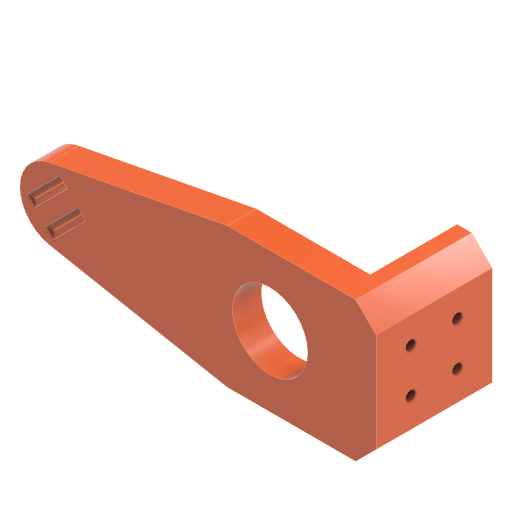
# Autodesk Inventor part: Corner Z Axis Carriage
Saved by Autodesk Inventor 2023.2 (Build 272271000, 271)
## iProperties
Created: 2023-02-17
Part Number: Corner Z Axis Carriage
Material: ABS Plastic
Document SubType Name: Modeling
Designer: remop
Density: 1.06 g/cm^3
Appearance: Smooth - Light Orange
Author: remop
Autodesk Inventor part; units mm, degrees
ref_plane "YZ Plane" through (0, 0, 0) normal (1, 0, 0) x (0, 1, 0)
ref_plane "XZ Plane" through (0, 0, 0) normal (0, 1, 0) x (-1, 0, 0)
ref_plane "XY Plane" through (0, 0, 0) normal (0, 0, 1) x (1, 0, 0)
sketch "Sketch1" plane through (0, 0, 0) normal (0, 0, 1) x (1, 0, 0)
  arc A0 (18.184259, -16.532371) -> (18.761762, -13.100955) centre (16.062938, -14.41105) ccw
  arc A1 (18.761762, 13.100955) -> (18.761762, -13.100955) centre (45.75, 0) ccw
  arc A2 (18.761762, 13.100955) -> (18.184259, 16.532371) centre (16.062938, 14.41105) ccw
  line L0 (11.532371, 23.184259) -> (18.184259, 16.532371)
  arc A3 (11.532371, 23.184259) -> (8.100955, 23.761762) centre (9.41105, 21.062938) ccw
  arc A4 (-18.100955, 23.761762) -> (8.100955, 23.761762) centre (-5, 50.75) ccw
  arc A5 (-18.100955, 23.761762) -> (-21.532371, 23.184259) centre (-19.41105, 21.062938) ccw
  line L1 (-28.184259, 16.532371) -> (-21.532371, 23.184259)
  arc A6 (-28.184259, 16.532371) -> (-28.761762, 13.100955) centre (-26.062938, 14.41105) ccw
  arc A7 (-28.761762, -13.100955) -> (-28.761762, 13.100955) centre (-55.75, 0) ccw
  arc A8 (-28.761762, -13.100955) -> (-28.184259, -16.532371) centre (-26.062938, -14.41105) ccw
  line L2 (-21.532371, -23.184259) -> (-28.184259, -16.532371)
  arc A9 (-21.532371, -23.184259) -> (-18.100955, -23.761762) centre (-19.41105, -21.062938) ccw
  arc A10 (8.100955, -23.761762) -> (-18.100955, -23.761762) centre (-5, -50.75) ccw
  arc A11 (8.100955, -23.761762) -> (11.532371, -23.184259) centre (9.41105, -21.062938) ccw
  line L3 (18.184259, -16.532371) -> (11.532371, -23.184259)
  circle A12 centre (10, -15) radius 4
  circle A13 centre (-20, -15) radius 4
  circle A14 centre (-20, 15) radius 4
  circle A15 centre (10, 15) radius 4
  circle A16 centre (-5, 0) radius 13
  line L4 (39.464466, -4.5) -> (34.964466, -4.5)
  line L5 (34.964466, -4.5) -> (34.964466, 4.5)
  line L6 (34.964466, 4.5) -> (39.464466, 4.5)
  line L7 (39.464466, 4.5) -> (39.464466, 10)
  line L8 (39.464466, 10) -> (31.464466, 10)
  line L9 (31.464466, 10) -> (31.464466, -10)
  line L10 (31.464466, -10) -> (39.464466, -10)
  line L11 (39.464466, -10) -> (39.464466, -4.5)
  line L12 (31.464466, -10) -> (31.464466, -17.071068)
  line L13 (31.464466, -17.071068) -> (24.472595, -24.062938)
  line L14 (31.464466, 10) -> (31.464466, 17.071068)
  line L15 (-19.41105, -24.062938) -> (24.472595, -24.062938)
  line L16 (-19.41105, 24.062938) -> (24.472595, 24.062938)
  line L17 (31.464466, 17.071068) -> (24.472595, 24.062938)
  circle A17 centre (-78.5, 0) radius 12.5
  line L18 (-19.978787, -24.008728) -> (-80.865571, -12.274122)
  line L19 (-80.865571, 12.274122) -> (-19.978787, 24.008728)
  point P0 (0, 0)
  dimension "d0" = 45
  dimension "d1" = 5
  dimension "d4" = 78.5
  dimension "d5" = 25
  constraints: 16 end point, 8 tangent, 6 point on circle, 3 equal length, 2 vertical, 1 centre point, 1 horizontal alignment, 1 point on line
  measures "d0" angle of L12 L13
  measures "d1" distance from line of L9.end L13
  measures "d4" distance of A17.centre point (0, 0)
  measures "d5" diameter of A17
extrude "Extrusion1" add sketch "Sketch1" along normal blind 10 contours L3 A11 A10 A9 L2 A8 A7 A6 L1 A5 A4 A3 L0 A2 A1 A0 | A0 A1 A2 L0 A3 L16 L17 L14 L9 L12 L13 L15 A11 L3 | L15 A9 A10 A11 | L18 A17 L19 A5 L1 A6 A7 A8 L2 A9 | A3 A4 A5 L16 | A17 | A12 | A14
sketch "Sketch2" plane through (0, 0, 0) normal (0, 0, -1) x (-1, 0, 0)
  line L0 (-24.472595, -24.062938) -> (-31.464466, -17.071068)
  line L1 (19.41105, -24.062938) -> (-24.472595, -24.062938)
  arc A0 (19.41105, -24.062938) -> (19.978787, -24.008728) centre (19.41105, -21.062938) ccw
  line L2 (80.865571, -12.274122) -> (19.978787, -24.008728)
  arc A1 (80.865571, -12.274122) -> (80.865571, 12.274122) centre (78.5, 0) ccw
  line L3 (19.978787, 24.008728) -> (80.865571, 12.274122)
  arc A2 (19.978787, 24.008728) -> (19.41105, 24.062938) centre (19.41105, 21.062938) ccw
  line L4 (-24.472595, 24.062938) -> (19.41105, 24.062938)
  line L5 (-31.464466, 17.071068) -> (-24.472595, 24.062938)
  line L6 (-31.464466, -17.071068) -> (-31.464466, 17.071068)
  circle A3 centre (20, -15) radius 4
  circle A4 centre (-10, 15) radius 4
  circle A5 centre (5, 0) radius 13
  line L7 (-31.464466, 17.071068) -> (-23.464466, 17.071068)
  line L8 (-23.464466, 17.071068) -> (-23.464466, -17.071068)
  line L9 (-24.472595, -24.062938) -> (-31.464466, -17.071068)
  line L10 (-23.464466, -17.071068) -> (-31.464466, -17.071068)
  line L11 (-23.464466, 17.071068) -> (-19.472595, 21.062938)
  line L12 (-19.472595, 21.062938) -> (-19.472595, 24.062938)
  line L13 (-23.464466, -17.071068) -> (-19.472595, -21.062938)
  line L14 (-19.472595, -21.062938) -> (-19.472595, -24.062938)
  line L15 (19.41105, -24.062938) -> (-24.472595, -24.062938)
  point P0 (0, 0)
  dimension "d6" = 8
  dimension "d9" = 3
  constraints: 14 end point, 3 perpendicular, 3 point on line, 2 horizontal, 1 parallel, 1 vertical
  measures "d6" distance of L5.start L7.end
  measures "d9" distance of L11.end L12.end
extrude "Extrusion2" add sketch "Sketch2" along normal blind 29.9 contours L0 L10 L13 L14 L1 | L6 L7 L8 L10 | L5 L4 L12 L11 L7
sketch "Sketch3" plane through (23.464466, -17.071068, 0) normal (-1, 0, 0) x (0, 0, 1)
  line L0 (0, 34.142136) -> (0, 0)
  line L1 (0, 34.142136) -> (-29.9, 34.142136)
  line L2 (-29.9, 0) -> (-29.9, 34.142136)
  line L3 (0, 0) -> (-29.9, 0)
  point P0 (0, 17.071068)
  point P1 (-1.95, 25.015758)
  point P2 (-17.95, 25.015758)
  point P3 (-17.95, 10.015758)
  point P4 (-1.95, 10.015758)
  dimension "d10" = 15
  dimension "d11" = 16
  dimension "d12" = 11.95
  constraints: 2 horizontal alignment, 2 vertical alignment
  measures "d10" distance of point (-1.95, 10.016) point (-1.95, 25.016)
  measures "d11" distance of point (-17.95, 25.016) point (-1.95, 25.016)
  measures "d12" distance from line of L2 point (-17.95, 25.016)
hole "Hole1" at (23.464466, 7.94469, -1.95) at (23.464466, 7.94469, -17.95) at (23.464466, -7.05531, -17.95) at (23.464466, -7.05531, -1.95) direction (1, 0, 0) diameter 3.6 end through all counterbore diameter 6.5 counterbore depth 3.4 clearance for "Socket Head Cap Screw DIN EN ISO 4762" size "M3" standard "DIN"
sketch "Sketch4" plane through (0, 0, 0) normal (0, 0, -1) x (-1, 0, 0)
  circle A0 centre (5, 0) radius 13
  circle A1 centre (-10, 15) radius 4
  circle A2 centre (20, -15) radius 4
  line L0 (-19.472595, 24.062938) -> (-19.472595, 21.062938)
  line L1 (-19.472595, 21.062938) -> (-23.464466, 17.071068)
  line L2 (-23.464466, 17.071068) -> (-23.464466, 10.54469)
  line L3 (-23.464466, 10.54469) -> (-23.464466, 5.34469)
  line L4 (-23.464466, 5.34469) -> (-23.464466, -4.45531)
  line L5 (-23.464466, -4.45531) -> (-23.464466, -9.65531)
  line L6 (-23.464466, -9.65531) -> (-23.464466, -17.071068)
  line L7 (-23.464466, -17.071068) -> (-19.472595, -21.062938)
  line L8 (-19.472595, -21.062938) -> (-19.472595, -24.062938)
  line L9 (19.41105, -24.062938) -> (-19.472595, -24.062938)
  arc A3 (19.41105, -24.062938) -> (19.978787, -24.008728) centre (19.41105, -21.062938) ccw
  line L10 (80.865571, -12.274122) -> (19.978787, -24.008728)
  arc A4 (80.865571, -12.274122) -> (80.865571, 12.274122) centre (78.5, 0) ccw
  line L11 (19.978787, 24.008728) -> (80.865571, 12.274122)
  arc A5 (19.978787, 24.008728) -> (19.41105, 24.062938) centre (19.41105, 21.062938) ccw
  line L12 (-19.472595, 24.062938) -> (19.41105, 24.062938)
  line L13 (-19.472595, 21.062938) -> (-15.480725, 17.071068)
  line L14 (-15.480725, 17.071068) -> (-15.480725, -17.071068)
  line L15 (-15.480725, -17.071068) -> (-19.472595, -21.062938)
  line L16 (-23.464466, 17.071068) -> (-19.472595, 21.062938)
  point P0 (0, 0)
  constraints: 6 end point, 3 perpendicular, 1 vertical
extrude "Extrusion3" cut sketch "Sketch4" against normal blind 2 contours L13 L14 L15 L7 L6 L5 L4 L3 L2 L1
sketch "Sketch5" plane through (0, 0, 10) normal (0, 0, 1) x (1, 0, 0)
  line L0 (24.472595, -24.062938) -> (31.464466, -17.071068)
  line L1 (31.464466, -17.071068) -> (31.464466, 17.071068)
  line L2 (31.464466, 17.071068) -> (24.472595, 24.062938)
  line L3 (24.472595, 24.062938) -> (-19.41105, 24.062938)
  arc A0 (-19.41105, 24.062938) -> (-19.978787, 24.008728) centre (-19.41105, 21.062938) ccw
  line L4 (-19.978787, 24.008728) -> (-80.865571, 12.274122)
  arc A1 (-80.865571, 12.274122) -> (-80.865571, -12.274122) centre (-78.5, 0) ccw
  line L5 (-80.865571, -12.274122) -> (-19.978787, -24.008728)
  arc A2 (-19.978787, -24.008728) -> (-19.41105, -24.062938) centre (-19.41105, -21.062938) ccw
  line L6 (-19.41105, -24.062938) -> (24.472595, -24.062938)
  circle A3 centre (-20, -15) radius 4
  circle A4 centre (10, 15) radius 4
  circle A5 centre (-5, 0) radius 13
  line L7 (-88.753048, -1.06066) -> (-77.43934, 10.253048)
  line L8 (-77.43934, 10.253048) -> (-74.610913, 7.424621)
  line L9 (-74.610913, 7.424621) -> (-85.924621, -3.889087)
  line L10 (-85.924621, -3.889087) -> (-88.753048, -1.06066)
  line L11 (-82.389087, -7.424621) -> (-71.075379, 3.889087)
  line L12 (-71.075379, 3.889087) -> (-68.246952, 1.06066)
  line L13 (-68.246952, 1.06066) -> (-79.56066, -10.253048)
  line L14 (-79.56066, -10.253048) -> (-82.389087, -7.424621)
  point P0 (0, 0)
  dimension "d22" = 16
  dimension "d23" = 4
  dimension "d24" = 8
  dimension "d25" = 2.5
  dimension "d26" = 2.5
  constraints: 16 end point, 6 perpendicular, 4 point on line, 1 collinear, 1 parallel
  measures "d22" distance of L7.start L7.end
  measures "d23" distance of L7.end L8.end
  measures "d24" distance from line of L10 A1.centre
  measures "d25" distance from line of A1.centre L9
  measures "d26" distance from line of A1.centre L11
extrude "Extrusion4" cut sketch "Sketch5" against normal blind 1.5 contours L7 L8 L9 L10 | L11 L12 L13 L14
fillet "Fillet1" radius 2 4 edges at (-83.0962, 4.5962, 8.5) (-80.2678, 1.7678, 8.5) (-76.7322, -1.7678, 8.5) (-73.9038, -4.5962, 8.5)
sketch "Sketch6" plane through (0, 0, 0) normal (0, 0, -1) x (-1, 0, 0)
  line L0 (-19.472595, 21.062938) -> (-15.480725, 17.071068)
  line L1 (-15.480725, 17.071068) -> (-15.480725, -17.071068)
  line L2 (-15.480725, -17.071068) -> (-19.472595, -21.062938)
  line L3 (-19.472595, -21.062938) -> (-19.472595, -24.062938)
  line L4 (19.41105, -24.062938) -> (-19.472595, -24.062938)
  arc A0 (19.41105, -24.062938) -> (19.978787, -24.008728) centre (19.41105, -21.062938) ccw
  line L5 (80.865571, -12.274122) -> (19.978787, -24.008728)
  arc A1 (80.865571, -12.274122) -> (80.865571, 12.274122) centre (78.5, 0) ccw
  line L6 (19.978787, 24.008728) -> (80.865571, 12.274122)
  arc A2 (19.978787, 24.008728) -> (19.41105, 24.062938) centre (19.41105, 21.062938) ccw
  line L7 (-19.472595, 24.062938) -> (19.41105, 24.062938)
  line L8 (-19.472595, 24.062938) -> (-19.472595, 21.062938)
  circle A3 centre (20, -15) radius 4
  circle A4 centre (-10, 15) radius 4
  circle A5 centre (5, 0) radius 13
  line L9 (26.717514, -18.889087) -> (16.110913, -8.282486)
  line L10 (16.110913, -8.282486) -> (18.232233, -6.161165)
  line L11 (18.232233, -6.161165) -> (28.838835, -16.767767)
  line L12 (28.838835, -16.767767) -> (26.717514, -18.889087)
  line L13 (13.282486, -11.110913) -> (23.889087, -21.717514)
  line L14 (23.889087, -21.717514) -> (21.767767, -23.838835)
  line L15 (21.767767, -23.838835) -> (11.161165, -13.232233)
  line L16 (11.161165, -13.232233) -> (13.282486, -11.110913)
  line L17 (26.717514, -18.889087) -> (23.889087, -21.717514) construction
  line L18 (20, -15) -> (21.414214, -13.585786) construction
  line L19 (20, -15) -> (18.585786, -16.414214) construction
  line L20 (-16.717514, 18.889087) -> (-6.110913, 8.282486)
  line L21 (-8.232233, 6.161165) -> (-18.838835, 16.767767)
  line L22 (-6.110913, 8.282486) -> (-8.232233, 6.161165)
  line L23 (-18.838835, 16.767767) -> (-16.717514, 18.889087)
  line L24 (-13.889087, 21.717514) -> (-11.767767, 23.838835)
  line L25 (-3.282486, 11.110913) -> (-13.889087, 21.717514)
  line L26 (-11.767767, 23.838835) -> (-1.161165, 13.232233)
  line L27 (-1.161165, 13.232233) -> (-3.282486, 11.110913)
  point P0 (0, 0)
  point P1 (-11.414214, 13.585786)
  point P2 (-8.585786, 16.414214)
  point P3 (-10.577657, 24.062938)
  point P4 (-11.543663, 24.062938)
  point P5 (-6.136297, 13.964724)
  point P6 (-11.035276, 18.863703)
  point P7 (-8.964724, 11.136297)
  point P8 (-13.863703, 16.035276)
  point P9 (21.621133, -23.692201)
  point P10 (21.984415, -23.622187)
  point P11 (21.035276, -18.863703)
  point P12 (16.136297, -13.964724)
  point P13 (23.863703, -16.035276)
  point P14 (18.964724, -11.136297)
  point P15 (-15.947469, 17.537812)
  point P16 (-15.480725, 12.347702)
  point P17 (18.456337, -24.062938)
  point P18 (19.422364, -24.062917)
  point P19 (-15.480725, 13.409657)
  point P20 (-17.008129, 18.598472)
  dimension "d30" = 45
  dimension "d31" = 3
  dimension "d32" = 4
  dimension "d33" = 15
  dimension "d36" = 360
  constraints: 38 end point, 4 parallel, 4 perpendicular, 3 equal length, 3 midpoint, 1 collinear, 1 point on line, 37 other
  measures "d30" angle of L4 L15
  measures "d31" distance of L11.end L9.start
  measures "d32" distance of L9.start L13.end
  measures "d33" distance of L10.end L11.end
extrude "Extrusion5" cut sketch "Sketch6" against normal blind 1.5 contours L23 L20 A4 L22 L21 L1 L0 | L0 L1 L21 L23 | L20 A4 | A4 L25 L20 | L25 L24 L26 L27 A4 | A4 L25 | L14 L15 L5 | L5 L15 L16 L13 A3 L14 | L13 A3 L9 | A3 L13 | L9 A3 | A3 L9 L10 L11 L12 | A5
fillet "Fillet4" radius 1 8 edges at (-18.9647, -11.1363, 0.75) (-16.1363, -13.9647, 0.75) (-21.0353, -18.8637, 0.75) (-23.8637, -16.0353, 0.75) (8.9647, 11.1363, 0.75) (6.1363, 13.9647, 0.75) (11.0353, 18.8637, 0.75) (13.8637, 16.0353, 0.75)
sketch "Sketch7" plane through (0, 0, 10) normal (0, 0, 1) x (1, 0, 0)
  circle A0 centre (10, 15) radius 4 projected
  circle A1 centre (-20, -15) radius 4 projected
  point P0 (0, 0)
extrude "Extrusion6" add sketch "Sketch7" against normal blind 3
fillet "Fillet5" radius 1.5 16 edges at (6.4645, 18.5355, 1.5) (11.8565, 9.7854, 1.5) (-23.5355, -11.4645, 1.5) (-16.3911, -18.4622, 1.5) (-15.9293, -13.2379, 1.5) (-14.2021, -12.0305, 1.5) (-21.7621, -19.0707, 1.5) (-22.9695, -20.7979, 1.5) (12.9695, 20.7979, 1.5) (11.7621, 19.0707, 1.5) (15.7979, 17.9695, 1.5) (14.0707, 16.7621, 1.5) (8.2379, 10.9293, 1.5) (7.0305, 9.2021, 1.5) (4.2021, 12.0305, 1.5) (5.9293, 13.2379, 1.5)
sketch "Sketch9" plane through (0, 0, 0) normal (0, 0, -1) x (-1, 0, 0)
  circle A0 centre (5, 0) radius 13
  arc A1 (-14.695015, 16.905158) -> (-13.336967, 17.205596) centre (-14.171208, 17.756995) ccw
  arc A2 (-12.205596, 18.336967) -> (-13.336967, 17.205596) centre (-10, 15) ccw
  arc A3 (-12.205596, 18.336967) -> (-12.049888, 19.878315) centre (-12.756995, 19.171208) ccw
  line L0 (-12.049888, 19.878315) -> (-13.889087, 21.717514)
  line L1 (-13.889087, 21.717514) -> (-11.767767, 23.838835)
  line L2 (-11.767767, 23.838835) -> (-1.161165, 13.232233)
  line L3 (-1.161165, 13.232233) -> (-3.282486, 11.110913)
  line L4 (-3.282486, 11.110913) -> (-5.121685, 12.950112)
  arc A4 (-5.121685, 12.950112) -> (-6.663033, 12.794404) centre (-5.828792, 12.243005) ccw
  arc A5 (-7.794404, 11.663033) -> (-6.663033, 12.794404) centre (-10, 15) ccw
  arc A6 (-7.794404, 11.663033) -> (-7.950112, 10.121685) centre (-7.243005, 10.828792) ccw
  line L5 (-7.950112, 10.121685) -> (-6.110913, 8.282486)
  line L6 (-6.110913, 8.282486) -> (-8.232233, 6.161165)
  line L7 (-8.232233, 6.161165) -> (-15.480725, 13.409657)
  line L8 (-15.480725, 13.409657) -> (-15.480725, -17.071068)
  line L9 (-15.480725, -17.071068) -> (-19.472595, -21.062938)
  line L10 (-19.472595, -21.062938) -> (-19.472595, -24.062938)
  line L11 (19.41105, -24.062938) -> (-19.472595, -24.062938)
  arc A7 (19.41105, -24.062938) -> (19.978787, -24.008728) centre (19.41105, -21.062938) ccw
  line L12 (21.621133, -23.692201) -> (19.978787, -24.008728)
  line L13 (21.621133, -23.692201) -> (11.161165, -13.232233)
  line L14 (11.161165, -13.232233) -> (13.282486, -11.110913)
  line L15 (13.282486, -11.110913) -> (15.121685, -12.950112)
  arc A8 (15.121685, -12.950112) -> (16.663033, -12.794404) centre (15.828792, -12.243005) ccw
  arc A9 (17.794404, -11.663033) -> (16.663033, -12.794404) centre (20, -15) ccw
  arc A10 (17.794404, -11.663033) -> (17.950112, -10.121685) centre (17.243005, -10.828792) ccw
  line L16 (17.950112, -10.121685) -> (16.110913, -8.282486)
  line L17 (16.110913, -8.282486) -> (18.232233, -6.161165)
  line L18 (18.232233, -6.161165) -> (28.838835, -16.767767)
  line L19 (28.838835, -16.767767) -> (26.717514, -18.889087)
  line L20 (26.717514, -18.889087) -> (24.878315, -17.049888)
  arc A11 (24.878315, -17.049888) -> (23.336967, -17.205596) centre (24.171208, -17.756995) ccw
  arc A12 (22.205596, -18.336967) -> (23.336967, -17.205596) centre (20, -15) ccw
  arc A13 (22.205596, -18.336967) -> (22.049888, -19.878315) centre (22.756995, -19.171208) ccw
  line L21 (22.049888, -19.878315) -> (23.889087, -21.717514)
  line L22 (23.889087, -21.717514) -> (21.984415, -23.622187)
  line L23 (80.865571, -12.274122) -> (21.984415, -23.622187)
  arc A14 (80.865571, -12.274122) -> (80.865571, 12.274122) centre (78.5, 0) ccw
  line L24 (19.978787, 24.008728) -> (80.865571, 12.274122)
  arc A15 (19.978787, 24.008728) -> (19.41105, 24.062938) centre (19.41105, 21.062938) ccw
  line L25 (-19.472595, 24.062938) -> (19.41105, 24.062938)
  line L26 (-19.472595, 24.062938) -> (-19.472595, 21.062938)
  line L27 (-19.472595, 21.062938) -> (-17.008129, 18.598472)
  line L28 (-17.008129, 18.598472) -> (-16.717514, 18.889087)
  line L29 (-16.717514, 18.889087) -> (-14.878315, 17.049888)
  arc A16 (-14.878315, 17.049888) -> (-14.695015, 16.905158) centre (-14.171208, 17.756995) ccw
  line L30 (40, 9.966046) -> (23.930249, 13.063142)
  line L31 (26.764312, 12.516938) -> (40, 9.966046)
  line L32 (40, -9.966046) -> (40, 9.966046)
  line L33 (40, 9.966046) -> (40, -9.966046)
  line L34 (40, -9.966046) -> (30.868148, -11.726012)
  line L35 (30.868148, -11.726012) -> (25.976757, -6.834621)
  circle A17 centre (5, 0) radius 23
  line L36 (80.865571, -12.274122) -> (21.984415, -23.622187)
  line L37 (50, -8.038763) -> (50, 8.038763)
  line L38 (50, 8.038763) -> (75.5, 3.124192)
  line L39 (75.5, 3.124192) -> (75.5, -3.124192)
  line L40 (75.5, -3.124192) -> (50, -8.038763)
  point P0 (0, 0)
  point P1 (26.716886, -7.574751)
  dimension "d49" = 10
  dimension "d50" = 5
  dimension "d51" = 10
  dimension "d52" = 10
  dimension "d53" = 35
  dimension "d54" = 10
  dimension "d55" = 10
  dimension "d56" = 10
  dimension "d57" = 3
  constraints: 20 end point, 6 parallel, 2 collinear, 2 vertical, 1 coincident, 1 point on line, 3 other
  measures "d50" distance between parallel lines of L18 L35
  measures "d51" distance between parallel lines of L23 L34
  measures "d52" distance between parallel lines of L24 L30
  measures "d53" distance from line of A0.centre L32
  measures "d54" distance between parallel lines of L23 L40
  measures "d55" distance between parallel lines of L24 L38
  measures "d56" distance between parallel lines of L37 L32
  measures "d57" distance from line of A14.centre L39
extrude "Extrusion7" cut sketch "Sketch9" against normal blind 7 contours L30 L32 L34 L35 A17 | L37 L38 L39 L40
fillet "Fillet6" radius 2 9 edges at (-75.5, 3.1242, 3.5) (-75.5, -3.1242, 3.5) (-50, -8.0388, 3.5) (-50, 8.0388, 3.5) (-40, -9.966, 3.5) (-30.8681, -11.726, 3.5) (-26.7169, -7.5748, 3.5) (-23.9302, 13.0631, 3.5) (-40, 9.966, 3.5)
chamfer "Chamfer1" distance 3 angle 45 18 edges at (-50, 0, 0) (-50.7266, 7.1587, 0) (-63.1285, 5.5085, 0) (-75.0422, 2.7462, 0) (-75.5, 0, 0) (-75.0422, -2.7462, 0) (-63.1285, -5.5085, 0) (-50.7266, -7.1587, 0) (-40, 0, 0) (-39.5422, -9.5881, 0) (-35.1444, -10.9019, 0) (-30.9456, -11.4734, 0) (-28.8484, -9.7062, 0) (-27.0557, -7.5182, 0) (-27.9443, 1.599, 0) (-26.218, 11.5228, 0) (-33.2721, 11.2627, 0) (-39.5422, 9.5881, 0)
equation "\"d24\" = 0.5 * d22"
equation "\"d26\" = d25"
equation "\"d51\" = d49"
equation "\"d52\" = d49"
equation "\"d54\" = d51"
equation "\"d55\" = d52"
equation "\"d56\" = d52"
body "Solid1"
